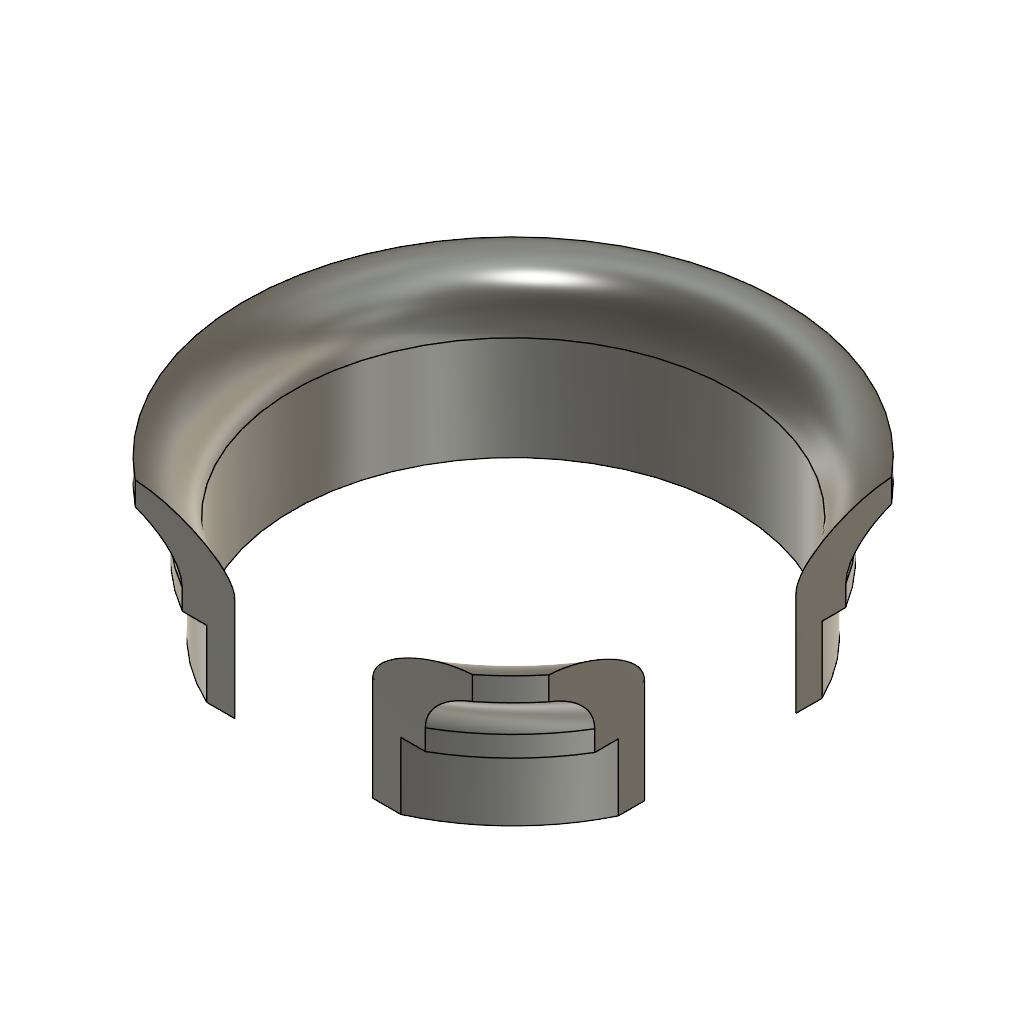
Port Back (Autodesk Fusion 360 design; units mm, degrees)
Autodesk Fusion 360 part; units mm, degrees
sketch "Sketch1" plane through (0, 0, 0) normal (0, 0, 1) x (1, 0, 0)
  circle A0 centre (0, 0) radius 33
  circle A1 centre (0, 0) radius 36.25
  dimension "d1" = 66
  dimension "d2" = 3.25
  constraint coincident A0.centre A1.centre
  measures "d1" diameter of A0
extrude "Extrude1" add sketch "Sketch1" along normal blind 10 makes body 1
sketch "Sketch2" plane through (0, 0, 10) normal (0, 0, 1) x (-1, 0, 0)
  circle A0 centre (0, 0) radius 33
  circle A1 centre (0, 0) radius 36.25
  circle A2 centre (0, 0) radius 33
  circle A3 centre (0, 0) radius 40.25
  dimension "d5" = 80.5
  constraint coincident A0.centre A1.centre
  constraint concentric A2 A3
  measures "d5" diameter of A3
extrude "Extrude2" add sketch "Sketch2" along normal blind 3.5 contours A1 | A3 bodies 1
fillet "Fillet1" radius 8 1 edges at (-33.7969, -13.1086, 10) on bodies 1
ref_plane "WorkPlane1" through (0, 0, 13.5) normal (0, 0, 1) x (-1, 0, 0)
fillet "Fillet2" radius 8 1 edges at (30.7668, -11.9333, 13.5) on bodies 1
sketch "Sketch5" plane through (0, 0, 0) normal (0, 0, -1) x (1, 0, 0)
  circle A0 centre (0, 0) radius 33
  circle A1 centre (0, 0) radius 36.25
  line L0 (0, 33) -> (0, 31.35)
  line L1 (0, 31.35) -> (45.3638, 31.35)
  line L2 (45.3638, 31.35) -> (45.3638, 44.0019)
  line L3 (45.3638, 44.0019) -> (-46.5761, 44.0019)
  line L4 (-46.5761, 44.0019) -> (-46.5761, 31.35)
  line L5 (-46.5761, 31.35) -> (0, 31.35)
  dimension "d13" = 1.65
  constraint coincident A0 L0.start
  constraint vertical L0
  constraint perpendicular L0 L1
  constraint perpendicular L1 L2
  constraint perpendicular L0 L3
  constraint perpendicular L1 L4
  constraint perpendicular L0 L5
  measures "d13" distance of L0.start L0.end
extrude "Extrude3" cut sketch "Sketch5" against normal blind 32 contours A0 L0 L1 | A0 A1 L1 L5 | A0 L0 L5 | A1 L1 L2 L3 L4 L5 picked at (11.2202, 33.2731) bodies 1
sketch "Sketch6" plane through (0, 0, 0) normal (0, 0, -1) x (1, 0, 0)
  line L0 (-10.3042, 31.35) -> (-18.2, 31.35)
  arc A0 (-18.2, 31.35) -> (18.2, 31.35) centre (0, 0) ccw
  line L1 (18.2, 31.35) -> (10.3042, 31.35)
  arc A1 (-10.3042, 31.35) -> (10.3042, 31.35) centre (0, 0) ccw
  circle A2 centre (0, 0) radius 33
  circle A3 centre (0, 0) radius 34.55
  line L2 (-10.3042, 31.35) -> (-14.2521, 31.35)
  line L3 (14.2521, 31.35) -> (10.3042, 31.35)
  dimension "d16" = 1.55
  constraint concentric A0 A2
  constraint coincident L0.start A1.start
  constraint midpoint L0 L2.end
  constraint midpoint L1 L3.start
  constraint coincident L1.end A1.end
extrude "Extrude4" add sketch "Sketch6" along normal blind 10 contours L0 L1 A1 A2 A3 L2 L3 bodies 1
sketch "Sketch7" plane through (0, 0, -10) normal (0, 0, -1) x (1, 0, 0)
  line L0 (-10.3042, 31.35) -> (-14.5217, 31.35)
  arc A0 (-14.5217, 31.35) -> (14.5217, 31.35) centre (0, 0) ccw
  line L1 (14.5217, 31.35) -> (10.3042, 31.35)
  arc A1 (-10.3042, 31.35) -> (10.3042, 31.35) centre (0, 0) ccw
  line L2 (33, 0) -> (31, 0)
  line L3 (31, 0) -> (31, -37.4243)
  line L4 (31, -37.4243) -> (46.2157, -37.4243)
  line L5 (46.2157, -37.4243) -> (46.2157, 36.2205)
  line L6 (46.2157, 36.2205) -> (31, 36.2205)
  line L7 (31, 36.2205) -> (31, -37.4243)
  dimension "d19" = 2
  constraint coincident A1 L2.start
  constraint horizontal L2
  constraint perpendicular L2 L3
  constraint horizontal L4
  constraint vertical L5
  constraint horizontal L6
  constraint vertical L7
  measures "d19" distance of L2.start L2.end
extrude "Extrude5" cut sketch "Sketch7" against normal blind 50 contours A1 L2 L3 L7 | A0 A1 L3 L7 | A0 L3 L4 L5 L6 L7 | A1 L2 L7 bodies 1 makes body 2 at (30.4848, -12.6363, -3.3333)
equation "d5 = 72.5 mm + 8 mm"
